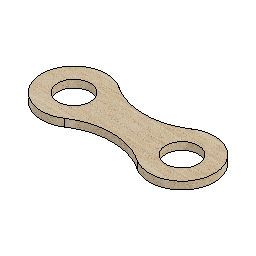
model (Autodesk Fusion 360 design; units mm, degrees)
Autodesk Fusion 360 part; units mm, degrees
sketch "Sketch1" plane through (0, 0, 0) normal (0, 0, 1) x (1, 0, 0) in component "clamp"
  circle A0 centre (60, 60) radius 27
  circle A1 centre (240, 60) radius 27
  arc A2 (210.2752, 14.9174) -> (89.7248, 14.9174) centre (150, -76.5) ccw
  arc A3 (89.7248, 105.0826) -> (210.2752, 105.0826) centre (150, 196.5) ccw
  arc A4 (89.7248, 105.0826) -> (89.7248, 14.9174) centre (60, 60) ccw
  arc A5 (210.2752, 14.9174) -> (210.2752, 105.0826) centre (240, 60) ccw
  dimension "d1" = 54
  dimension "d2" = 54
  dimension "d6" = 180
  dimension "d9" = 54
  dimension "d10" = 54
  constraint tangent A3 A4
  constraint tangent A3 A5
  constraint coincident A2.end A4.end
  constraint coincident A2.start A5.start
  constraint tangent A2 A4
  constraint tangent A2 A5
  measures "d1" diameter of A0
  measures "d2" diameter of A1
  measures "d6" distance of A0.centre A1.centre
  measures "d9" radius of A5
  measures "d10" radius of A4
extrude "Extrude1" add sketch "Sketch1" along normal blind 13 makes body 1 in component "clamp"
extrude "Extrude1'" add sketch "Sketch1" along normal blind 12.7 separate body makes body 2
component "clamp" placed x (1, 0, 0) y (0, 1, 0) z (0, 0, 1) at (0, 0, 0)
hidden bodies 1
equation "d2 = d1"
equation "d9 = d1"
equation "d10 = d1"
equation "d17 = 1/2\""
